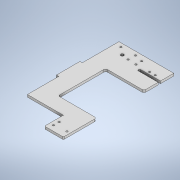
# Autodesk Inventor part: BAttery divider
Saved by Autodesk Inventor 2021 (Build 250183000, 183)
## iProperties
Created: 2020-08-12
Part Number: BAttery divider
Material: Generic
Document SubType Name: Modeling
Designer: jgray
Density: 1 g/cm^3
Appearance: Default
Author: jgray
Autodesk Inventor part; units mm, degrees
ref_plane "YZ Plane" through (0, 0, 0) normal (1, 0, 0) x (0, 1, 0)
ref_plane "XZ Plane" through (0, 0, 0) normal (0, 1, 0) x (-1, 0, 0)
ref_plane "XY Plane" through (0, 0, 0) normal (0, 0, 1) x (1, 0, 0)
sketch "Sketch1" plane through (0, 0, 0) normal (0, 1, 0) x (-1, 0, 0)
  line L0 (40, -5) -> (116.2, -5)
  line L1 (116.2, -199) -> (0, -199)
  line L2 (0, -199) -> (0, 0)
  line L3 (40, -5) -> (40, 35)
  line L4 (40, 35) -> (0, 35)
  line L5 (0, 35) -> (0, 0)
  line L6 (116.2, -71.25) -> (121.2, -71.25)
  line L7 (121.2, -71.25) -> (121.2, -121.25)
  line L8 (121.2, -121.25) -> (116.2, -121.25)
  line L9 (116.2, -5) -> (116.2, -71.25)
  line L10 (116.2, -121.25) -> (116.2, -199)
  dimension "d0" = 116.2
  dimension "d6" = 77.75
  dimension "d8" = 50
  dimension "d9" = 5
  dimension "d11" = 40
  dimension "d12" = 40
  dimension "d31" = 194
  constraints: 22 end point, 5 parallel, 3 perpendicular, 2 collinear, 2 horizontal
  measures "d0" distance of L1.start L1.end
  measures "d6" distance between parallel lines of L1 L8
  measures "d8" distance of L6.end L7.end
  measures "d9" distance of L7.end L8.end
  measures "d11" distance of L0.start L3.end
  measures "d12" distance of L3.end L4.end
  measures "d31" distance between parallel lines of L1 L0
extrude "Extrusion1" add sketch "Sketch1" along normal blind 5
sketch "Sketch2" plane through (0, 5, 0) normal (0, 1, 0) x (1, 0, 0)
  line L0 (-32, -64.6005) -> (-32, 40.6005) construction
  line L1 (-139.7989, 191) -> (-75.0444, 191) construction
  line L2 (0, 199) -> (-116.2, 199) projected
  line L3 (-116.2, 199) -> (-116.2, 121.25) projected
  line L4 (-116.2, 5) -> (-40, 5) projected
  line L5 (-40, 5) -> (-40, -35) projected
  point P0 (0, 0)
  point P1 (-32, -24)
  point P2 (-32, -12)
  point P3 (-104.2, 191)
  point P4 (-73.2, 191)
  point P5 (-32, -12)
  dimension "d16" = 31
  dimension "d17" = 8
  dimension "d18" = 12
  dimension "d19" = 17
  dimension "d20" = 12
  dimension "d21" = 8
  constraints: 4 end point, 3 point on line, 1 coincident, 1 horizontal, 1 midpoint, 1 vertical
  measures "d16" distance of point (-73.2, 191) point (-104.2, 191)
  measures "d17" distance between parallel lines of L2 L1
  measures "d18" distance from line of L3 point (-104.2, 191)
  measures "d19" distance from line of L4 point (-32, -12)
  measures "d20" distance of point (-32, -12) point (-32, -24)
  measures "d21" distance between parallel lines of L0 L5
hole "Hole1" at (-32, 5, 24) at (-32, 5, 12) at (-104.2, 5, -191) at (-73.2, 5, -191) direction (0, -1, 0) diameter 3.8 end through all
fillet "Fillet1" radius 2 2 edges at (-40, 2.5, 35) (0, 2.5, 35)
sketch "Sketch3" plane through (0, 5, 0) normal (0, 1, 0) x (1, 0, 0)
  line L0 (-56.2, 96.1981) -> (-56.2, 272.5509) construction
  line L1 (-116.2, 199) -> (-116.2, 121.25) projected
  line L2 (0, 199) -> (-116.2, 199) projected
  point P0 (0, 0)
  point P1 (-56.2, 187)
  point P2 (-56.2, 175)
  dimension "d32" = 60
  dimension "d33" = 12
  dimension "d34" = 12
  constraints: 2 end point, 2 point on line, 1 vertical
  measures "d32" distance between parallel lines of L1 L0
  measures "d33" distance from line of L2 point (-56.2, 187)
  measures "d34" distance of point (-56.2, 187) point (-56.2, 175)
hole "Hole2" at (-56.2, 5, -187) at (-56.2, 5, -175) direction (0, -1, 0) diameter 3.8 end through all
sketch "Sketch5" plane through (0, 5, 0) normal (0, 1, 0) x (1, 0, 0)
  line L0 (0, -33) -> (0, 199) projected
  line L1 (0, 170.75) -> (-42, 170.75)
  line L2 (-44, 168.75) -> (-44, 167.7)
  line L3 (-42, 165.7) -> (0, 165.7)
  line L4 (0, 165.7) -> (0, 170.75)
  line L5 (0, 199) -> (-116.2, 199) projected
  arc A0 (-44, 167.7) -> (-42, 165.7) centre (-42, 167.7) ccw
  arc A1 (-42, 170.75) -> (-44, 168.75) centre (-42, 168.75) ccw
  point P0 (0, 0)
  point P1 (-44, 165.7)
  point P2 (-44, 170.75)
  point P3 (0, 165.7)
  dimension "d47" = 44
  dimension "d48" = 5.05
  dimension "d49" = 33.3
  dimension "d50" = 2
  constraints: 8 end point, 5 point on line, 4 point on circle, 4 tangent, 2 centre point, 2 parallel, 1 equal radius, 1 horizontal, 1 perpendicular
  measures "d47" distance of L3.end point (-44, 165.7)
  measures "d48" distance of point (-44, 165.7) point (-44, 170.75)
  measures "d49" distance between parallel lines of L5 L3
  measures "d50" radius of A0
extrude "Extrusion3" cut sketch "Sketch5" against normal blind 5
sketch "Sketch6" plane through (0, 5, 0) normal (0, 1, 0) x (1, 0, 0)
  line L0 (-135.5788, 175.75) -> (79.5788, 175.75) construction
  line L1 (0, 199) -> (-116.2, 199) construction
  line L2 (0, 170.75) -> (0, 199) construction
  point P0 (0, 0)
  point P1 (-16, 175.75)
  point P2 (-28, 175.75)
  point P3 (-73.5, 175.75)
  dimension "d53" = 23.25
  dimension "d54" = 16
  dimension "d55" = 28
  dimension "d56" = 73.5
  constraints: 2 end point, 2 point on line, 1 horizontal, 1 midpoint
  measures "d53" distance between parallel lines of L1 L0
  measures "d54" distance from line of L2 point (-16, 175.75)
  measures "d55" distance from line of point (-28, 175.75) L2
  measures "d56" distance from line of point (-73.5, 175.75) L2
hole "Hole3" at (-16, 5, -175.75) at (-28, 5, -175.75) at (-73.5, 5, -175.75) direction (0, -1, 0) diameter 3.8 end through all
sketch "Sketch7" plane through (0, 5, 0) normal (0, 1, 0) x (1, 0, 0)
  line L0 (-6.5, 43.9272) -> (-6.5, -51.0616) construction
  line L1 (0, -33) -> (0, 165.7) projected
  line L2 (-38, -35) -> (-2, -35) projected
  point P0 (0, 0)
  point P1 (-6.5, -21)
  dimension "d64" = 6.5
  dimension "d65" = 14
  constraints: 2 end point, 1 point on line, 1 vertical
  measures "d64" distance between parallel lines of L1 L0
  measures "d65" distance from line of L2 point (-6.5, -21)
hole "Hole4" at (-6.5, 5, 21) direction (0, -1, 0) diameter 3.8 end through all
sketch "Sketch8" plane through (0, 5, 0) normal (0, 1, 0) x (1, 0, 0)
  line L0 (-129.4929, 178) -> (-73.5, 178) construction
  line L1 (0, 199) -> (-116.2, 199) projected
  line L2 (-88.7, 175) -> (-87.7, 175)
  line L3 (-85.2, 177.5) -> (-85.2, 178.5)
  line L4 (-87.7, 181) -> (-88.7, 181)
  line L5 (-91.2, 178.5) -> (-91.2, 177.5)
  line L6 (-91.2, 175) -> (-85.2, 181) construction
  line L7 (-85.2, 175) -> (-91.2, 181) construction
  line L8 (-116.2, 199) -> (-116.2, 121.25) projected
  arc A0 (-88.7, 181) -> (-91.2, 178.5) centre (-88.7, 178.5) ccw
  arc A1 (-91.2, 177.5) -> (-88.7, 175) centre (-88.7, 177.5) ccw
  arc A2 (-87.7, 175) -> (-85.2, 177.5) centre (-87.7, 177.5) ccw
  arc A3 (-85.2, 178.5) -> (-87.7, 181) centre (-87.7, 178.5) ccw
  point P0 (0, 0)
  point P1 (-88.2, 178)
  dimension "d73" = 21
  dimension "d74" = 6
  dimension "d75" = 6
  dimension "d76" = 25
  dimension "d77" = 2.5
  constraints: 14 end point, 9 point on line, 8 point on circle, 8 tangent, 4 centre point, 3 equal radius, 2 horizontal, 2 midpoint, 2 parallel, 1 perpendicular
  measures "d73" distance between parallel lines of L0 L1
  measures "d74" distance of L7.end L6.end
  measures "d75" distance of L6.end L7.start
  measures "d76" distance between parallel lines of L8 L5
  measures "d77" radius of A0
extrude "Extrusion4" cut sketch "Sketch8" against normal through all
sketch "Sketch9" plane through (0, 5, 0) normal (0, 1, 0) x (1, 0, 0)
  line L0 (0, -33) -> (0, 165.7) projected
  line L1 (0, 135.7) -> (-81.2, 135.7)
  line L2 (-81.2, 135.7) -> (-81.2, 35)
  line L3 (-81.2, 35) -> (0, 35)
  line L4 (0, 35) -> (0, 135.7)
  line L5 (0, 165.7) -> (-42, 165.7) projected
  line L6 (-116.2, 5) -> (-40, 5) projected
  line L7 (-116.2, 199) -> (-116.2, 121.25) projected
  point P0 (0, 0)
  point P1 (0, 35)
  dimension "d80" = 30
  dimension "d81" = 30
  dimension "d82" = 35
  constraints: 8 end point, 2 parallel, 1 horizontal, 1 perpendicular, 1 point on line
  measures "d80" distance between parallel lines of L1 L5
  measures "d81" distance between parallel lines of L6 L3
  measures "d82" distance between parallel lines of L2 L7
extrude "Extrusion5" cut sketch "Sketch9" against normal through all
fillet "Fillet3" radius 4 4 edges at (-81.2, 2.5, -135.7) (-81.2, 2.5, -35) (0, 2.5, -35) (0, 2.5, -135.7)
body "Solid1"
